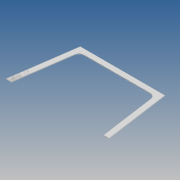
# Autodesk Inventor part: Cabine_Vitre_Avant_Haut
Saved by Autodesk Inventor 2019 (Build 230136000, 136)
## iProperties
Created: 2019-08-28
Part Number: Cabine_Vitre_Avant_Haut
Material: PVC-U
Document SubType Name: Modeling
Designer: jeremias.salamin
Density: 1.4 g/cm^3
Appearance: Lisse - Blanc
Description: Cabine Vitre Avant Haut
Author: jeremias.salamin
Autodesk Inventor part; units mm, degrees
ref_plane "YZ Plane" through (0, 0, 0) normal (1, 0, 0) x (0, 1, 0)
ref_plane "XZ Plane" through (0, 0, 0) normal (0, 1, 0) x (-1, 0, 0)
ref_plane "XY Plane" through (0, 0, 0) normal (0, 0, 1) x (1, 0, 0)
sketch "Sketch1" plane through (0, 0, 0) normal (0, 0, 1) x (1, 0, 0)
  line L0 (0, 60) -> (0, -80) construction
  line L1 (-110.88, 0) -> (110.88, 0) construction
  line L2 (-79.2, -60) -> (79.2, -60)
  line L3 (79.2, -60) -> (65, 40)
  line L4 (-65, 40) -> (65, 40)
  line L5 (-65, 40) -> (-79.2, -60)
  point P0 (0, 0)
  dimension "d0" = 158.4
  dimension "d9" = 130
  dimension "d10" = 60
  dimension "d11" = 100
  constraints: 8 end point, 2 horizontal, 1 symmetric about line, 1 other
  measures "d0" distance of L2.start L2.end
  measures "d9" distance of L4.start L3.end
  measures "d10" distance between parallel lines of L2 L1
  measures "d11" distance between parallel lines of L2 L4
extrude "Extrusion1" add sketch "Sketch1" along normal mid plane 0.8
sketch "Esquisse2" plane through (0, 0, 0.4) normal (0, 0, 1) x (1, 0, 0)
  line L0 (-79.2, -60) -> (79.2, -60) construction
  line L1 (79.2, -60) -> (65, 40) construction
  line L2 (65, 40) -> (-65, 40) construction
  line L3 (-65, 40) -> (-79.2, -60) construction
  line L4 (0, 60) -> (0, -80) construction
  line L5 (-110.88, 0) -> (110.88, 0) construction
  line L6 (-51.1115, 32) -> (51.1115, 32)
  line L7 (-59.032, 25.1247) -> (-71.1197, -60)
  line L8 (59.032, 25.1247) -> (71.1197, -60)
  arc A0 (-51.1115, 32) -> (-59.032, 25.1247) centre (-51.1115, 24) ccw
  arc A1 (59.032, 25.1247) -> (51.1115, 32) centre (51.1115, 24) ccw
  line L9 (-71.1197, -60) -> (71.1197, -60)
  point P0 (0, 0)
  dimension "d12" = 8
  dimension "d15" = 8
  dimension "d16" = 8
  constraints: 8 end point, 4 point on circle, 4 tangent, 3 parallel, 2 centre point, 2 point on line, 1 collinear, 1 equal radius, 1 horizontal, 1 other
  measures "d12" distance between parallel lines of L2 L6
  measures "d15" distance between parallel lines of L3 L7
  measures "d16" radius of A0
extrude "Extrusion2" cut sketch "Esquisse2" against normal through all
